Autodesk Fusion 360 part; units mm, degrees
note: some values were not read from the file. Set by a fixed rule: which face or edge a step refers to.
(part 3 of 3)
sketch "Skizze19" plane through (0, 0, 10) normal (0, 0, -1) x (1, 0, 0)
  circle A0 centre (420.5074, 124.379) radius 12
  circle A1 centre (87.5074, 162.379) radius 12
  circle A2 centre (120.8074, 162.379) radius 12
  circle A3 centre (154.1074, 162.379) radius 12
  circle A4 centre (187.4074, 162.379) radius 12
  circle A5 centre (220.7074, 162.379) radius 12
  circle A6 centre (254.0074, 162.379) radius 12
  circle A7 centre (287.3074, 162.379) radius 12
  circle A8 centre (320.6074, 162.379) radius 12
  circle A9 centre (353.9074, 162.379) radius 12
  circle A10 centre (387.2074, 162.379) radius 12
  circle A11 centre (420.5074, 162.379) radius 12
  line L0 (376.8151, 194.379) -> (364.2997, 194.379)
  arc A12 (343.5151, 194.379) -> (364.2997, 194.379) centre (353.9074, 200.379) ccw
  line L1 (343.5151, 194.379) -> (330.9997, 194.379)
  arc A13 (310.2151, 194.379) -> (330.9997, 194.379) centre (320.6074, 200.379) ccw
  line L2 (310.2151, 194.379) -> (297.6997, 194.379)
  arc A14 (276.9151, 194.379) -> (297.6997, 194.379) centre (287.3074, 200.379) ccw
  line L3 (276.9151, 194.379) -> (264.3997, 194.379)
  arc A15 (243.6151, 194.379) -> (264.3997, 194.379) centre (254.0074, 200.379) ccw
  line L4 (243.6151, 194.379) -> (231.0997, 194.379)
  arc A16 (210.3151, 194.379) -> (231.0997, 194.379) centre (220.7074, 200.379) ccw
  line L5 (210.3151, 194.379) -> (197.7997, 194.379)
  arc A17 (177.0151, 194.379) -> (197.7997, 194.379) centre (187.4074, 200.379) ccw
  line L6 (177.0151, 194.379) -> (164.4997, 194.379)
  arc A18 (143.7151, 194.379) -> (164.4997, 194.379) centre (154.1074, 200.379) ccw
  line L7 (143.7151, 194.379) -> (131.1997, 194.379)
  arc A19 (110.4151, 194.379) -> (131.1997, 194.379) centre (120.8074, 200.379) ccw
  line L8 (110.4151, 194.379) -> (97.8997, 194.379)
  arc A20 (77.1151, 194.379) -> (97.8997, 194.379) centre (87.5074, 200.379) ccw
  line L9 (77.1151, 194.379) -> (60.1074, 194.379)
  line L10 (60.1074, 194.379) -> (60.1074, 64.779)
  line L11 (60.1074, 64.779) -> (447.9074, 64.779)
  line L12 (447.9074, 64.779) -> (447.9074, 194.379)
  line L13 (447.9074, 194.379) -> (430.8997, 194.379)
  arc A21 (410.1151, 194.379) -> (430.8997, 194.379) centre (420.5074, 200.379) ccw
  line L14 (410.1151, 194.379) -> (397.5997, 194.379)
  arc A22 (376.8151, 194.379) -> (397.5997, 194.379) centre (387.2074, 200.379) ccw
  circle A23 centre (87.5074, 86.379) radius 12
  circle A24 centre (120.8074, 86.379) radius 12
  circle A25 centre (154.1074, 86.379) radius 12
  circle A26 centre (187.4074, 86.379) radius 12
  circle A27 centre (220.7074, 86.379) radius 12
  circle A28 centre (254.0074, 86.379) radius 12
  circle A29 centre (287.3074, 86.379) radius 12
  circle A30 centre (320.6074, 86.379) radius 12
  circle A31 centre (353.9074, 86.379) radius 12
  circle A32 centre (387.2074, 86.379) radius 12
  circle A33 centre (420.5074, 86.379) radius 12
  circle A34 centre (87.5074, 124.379) radius 12
  circle A35 centre (120.8074, 124.379) radius 12
  circle A36 centre (154.1074, 124.379) radius 12
  circle A37 centre (187.4074, 124.379) radius 12
  circle A38 centre (220.7074, 124.379) radius 12
  circle A39 centre (254.0074, 124.379) radius 12
  circle A40 centre (287.3074, 124.379) radius 12
  circle A41 centre (320.6074, 124.379) radius 12
  circle A42 centre (353.9074, 124.379) radius 12
  circle A43 centre (387.2074, 124.379) radius 12
  line L15 (60.1074, 168.379) -> (447.9074, 168.379)
  line L16 (447.9074, 168.379) -> (447.9074, 156.379)
  line L17 (447.9074, 156.379) -> (60.1074, 156.379)
  line L18 (60.1074, 156.379) -> (60.1074, 168.379)
  dimension "d256" = 6
  dimension "d257" = 6
  constraint horizontal L15
  constraint vertical L16
  constraint horizontal L17
  constraint vertical L18
  constraint collinear L10 L18
  constraint collinear L12 L16
  measures "d256" distance of A1.centre L15
  measures "d257" distance of A1.centre L17
extrude "Extrusion22" cut sketch "Skizze19" against normal blind 1 contours A1 A2 L15 L17 | A1 L10 L15 L17 L18 | A2 A3 L15 L17 | A3 A4 L15 L17 | A11 L12 L15 L16 L17 | A4 A5 L15 L17 | A10 A11 L15 L17 | A5 A6 L15 L17 | A9 A10 L15 L17 | A6 A7 L15 L17 | A8 A9 L15 L17 | A7 A8 L15 L17
sketch "Skizze20" plane through (0, 0, 10) normal (0, 0, -1) x (1, 0, 0)
  circle A0 centre (387.2074, 124.379) radius 12
  circle A1 centre (353.9074, 124.379) radius 12
  circle A2 centre (320.6074, 124.379) radius 12
  circle A3 centre (287.3074, 124.379) radius 12
  circle A4 centre (254.0074, 124.379) radius 12
  circle A5 centre (220.7074, 124.379) radius 12
  circle A6 centre (187.4074, 124.379) radius 12
  circle A7 centre (154.1074, 124.379) radius 12
  circle A8 centre (120.8074, 124.379) radius 12
  circle A9 centre (87.5074, 124.379) radius 12
  circle A10 centre (420.5074, 86.379) radius 12
  circle A11 centre (387.2074, 86.379) radius 12
  circle A12 centre (353.9074, 86.379) radius 12
  circle A13 centre (320.6074, 86.379) radius 12
  circle A14 centre (287.3074, 86.379) radius 12
  circle A15 centre (254.0074, 86.379) radius 12
  circle A16 centre (220.7074, 86.379) radius 12
  circle A17 centre (187.4074, 86.379) radius 12
  circle A18 centre (154.1074, 86.379) radius 12
  circle A19 centre (120.8074, 86.379) radius 12
  circle A20 centre (87.5074, 86.379) radius 12
  line L0 (376.8151, 156.379) -> (364.2997, 156.379)
  arc A21 (343.5151, 156.379) -> (364.2997, 156.379) centre (353.9074, 162.379) ccw
  line L1 (343.5151, 156.379) -> (330.9997, 156.379)
  arc A22 (310.2151, 156.379) -> (330.9997, 156.379) centre (320.6074, 162.379) ccw
  line L2 (310.2151, 156.379) -> (297.6997, 156.379)
  arc A23 (276.9151, 156.379) -> (297.6997, 156.379) centre (287.3074, 162.379) ccw
  line L3 (276.9151, 156.379) -> (264.3997, 156.379)
  arc A24 (243.6151, 156.379) -> (264.3997, 156.379) centre (254.0074, 162.379) ccw
  line L4 (243.6151, 156.379) -> (231.0997, 156.379)
  arc A25 (210.3151, 156.379) -> (231.0997, 156.379) centre (220.7074, 162.379) ccw
  line L5 (210.3151, 156.379) -> (197.7997, 156.379)
  arc A26 (177.0151, 156.379) -> (197.7997, 156.379) centre (187.4074, 162.379) ccw
  line L6 (177.0151, 156.379) -> (164.4997, 156.379)
  arc A27 (143.7151, 156.379) -> (164.4997, 156.379) centre (154.1074, 162.379) ccw
  line L7 (143.7151, 156.379) -> (131.1997, 156.379)
  arc A28 (110.4151, 156.379) -> (131.1997, 156.379) centre (120.8074, 162.379) ccw
  line L8 (110.4151, 156.379) -> (97.8997, 156.379)
  arc A29 (77.1151, 156.379) -> (97.8997, 156.379) centre (87.5074, 162.379) ccw
  line L9 (77.1151, 156.379) -> (60.1074, 156.379)
  line L10 (60.1074, 156.379) -> (60.1074, 64.779)
  line L11 (60.1074, 64.779) -> (447.9074, 64.779)
  line L12 (447.9074, 64.779) -> (447.9074, 156.379)
  line L13 (447.9074, 156.379) -> (430.8997, 156.379)
  arc A30 (410.1151, 156.379) -> (430.8997, 156.379) centre (420.5074, 162.379) ccw
  line L14 (410.1151, 156.379) -> (397.5997, 156.379)
  arc A31 (376.8151, 156.379) -> (397.5997, 156.379) centre (387.2074, 162.379) ccw
  circle A32 centre (420.5074, 124.379) radius 12
  line L15 (60.1074, 130.379) -> (447.9074, 130.379)
  line L16 (447.9074, 130.379) -> (447.9074, 118.379)
  line L17 (447.9074, 118.379) -> (60.1074, 118.379)
  line L18 (60.1074, 118.379) -> (60.1074, 130.379)
  dimension "d260" = 6
  dimension "d261" = 6
  constraint horizontal L15
  constraint vertical L16
  constraint horizontal L17
  constraint vertical L18
  constraint collinear L10 L18
  constraint collinear L12 L16
  measures "d260" distance of A9.centre L15
  measures "d261" distance of A9.centre L17
extrude "Extrusion23" cut sketch "Skizze20" against normal blind 1 contours A0 A32 L15 L17 | A0 A1 L15 L17 | L12 A32 L15 L16 L17 | A1 A2 L15 L17 | A2 A3 L15 L17 | A9 L10 L15 L17 L18 | A3 A4 L15 L17 | A8 A9 L15 L17 | A4 A5 L15 L17 | A7 A8 L15 L17 | A5 A6 L15 L17 | A6 A7 L15 L17
sketch "Skizze21" plane through (0, 0, 10) normal (0, 0, -1) x (1, 0, 0)
  circle A0 centre (87.5074, 86.379) radius 12
  circle A1 centre (120.8074, 86.379) radius 12
  circle A2 centre (154.1074, 86.379) radius 12
  circle A3 centre (187.4074, 86.379) radius 12
  circle A4 centre (220.7074, 86.379) radius 12
  circle A5 centre (254.0074, 86.379) radius 12
  circle A6 centre (287.3074, 86.379) radius 12
  circle A7 centre (320.6074, 86.379) radius 12
  circle A8 centre (353.9074, 86.379) radius 12
  circle A9 centre (387.2074, 86.379) radius 12
  circle A10 centre (420.5074, 86.379) radius 12
  line L0 (376.8151, 118.379) -> (364.2997, 118.379)
  arc A11 (343.5151, 118.379) -> (364.2997, 118.379) centre (353.9074, 124.379) ccw
  line L1 (343.5151, 118.379) -> (330.9997, 118.379)
  arc A12 (310.2151, 118.379) -> (330.9997, 118.379) centre (320.6074, 124.379) ccw
  line L2 (310.2151, 118.379) -> (297.6997, 118.379)
  arc A13 (276.9151, 118.379) -> (297.6997, 118.379) centre (287.3074, 124.379) ccw
  line L3 (276.9151, 118.379) -> (264.3997, 118.379)
  arc A14 (243.6151, 118.379) -> (264.3997, 118.379) centre (254.0074, 124.379) ccw
  line L4 (243.6151, 118.379) -> (231.0997, 118.379)
  arc A15 (210.3151, 118.379) -> (231.0997, 118.379) centre (220.7074, 124.379) ccw
  line L5 (210.3151, 118.379) -> (197.7997, 118.379)
  arc A16 (177.0151, 118.379) -> (197.7997, 118.379) centre (187.4074, 124.379) ccw
  line L6 (177.0151, 118.379) -> (164.4997, 118.379)
  arc A17 (143.7151, 118.379) -> (164.4997, 118.379) centre (154.1074, 124.379) ccw
  line L7 (143.7151, 118.379) -> (131.1997, 118.379)
  arc A18 (110.4151, 118.379) -> (131.1997, 118.379) centre (120.8074, 124.379) ccw
  line L8 (110.4151, 118.379) -> (97.8997, 118.379)
  arc A19 (77.1151, 118.379) -> (97.8997, 118.379) centre (87.5074, 124.379) ccw
  line L9 (77.1151, 118.379) -> (60.1074, 118.379)
  line L10 (60.1074, 118.379) -> (60.1074, 64.779)
  line L11 (60.1074, 64.779) -> (447.9074, 64.779)
  line L12 (447.9074, 64.779) -> (447.9074, 118.379)
  line L13 (447.9074, 118.379) -> (430.8997, 118.379)
  arc A20 (410.1151, 118.379) -> (430.8997, 118.379) centre (420.5074, 124.379) ccw
  line L14 (410.1151, 118.379) -> (397.5997, 118.379)
  arc A21 (376.8151, 118.379) -> (397.5997, 118.379) centre (387.2074, 124.379) ccw
  line L15 (60.1074, 92.379) -> (447.9074, 92.379)
  line L16 (447.9074, 92.379) -> (447.9074, 80.379)
  line L17 (447.9074, 80.379) -> (60.1074, 80.379)
  line L18 (60.1074, 80.379) -> (60.1074, 92.379)
  dimension "d264" = 6
  dimension "d265" = 6
  constraint horizontal L15
  constraint vertical L16
  constraint horizontal L17
  constraint vertical L18
  constraint collinear L10 L18
  constraint collinear L12 L16
  measures "d264" distance of A0.centre L15
  measures "d265" distance of A0.centre L17
extrude "Extrusion24" cut sketch "Skizze21" against normal blind 1 contours A0 A1 L15 L17 | A0 L10 L15 L17 L18 | A1 A2 L15 L17 | A2 A3 L15 L17 | A10 L12 L15 L16 L17 | A3 A4 L15 L17 | A9 A10 L15 L17 | A4 A5 L15 L17 | A8 A9 L15 L17 | A5 A6 L15 L17 | A7 A8 L15 L17 | A6 A7 L15 L17
sketch "Skizze22" plane through (0, 0, 30) normal (0, 0, 1) x (-1, 0, 0)
  circle A0 centre (-120.8074, 276.379) radius 12
  circle A1 centre (-87.5074, 276.379) radius 12
  circle A2 centre (-420.5074, 238.379) radius 12
  circle A3 centre (-387.2074, 238.379) radius 12
  circle A4 centre (-87.5074, 86.379) radius 12
  circle A5 centre (-28.1074, 23.779) radius 10.8095
  circle A6 centre (-479.9074, 23.779) radius 12
  circle A7 centre (-120.8074, 86.379) radius 12
  circle A8 centre (-154.1074, 86.379) radius 12
  circle A9 centre (-187.4074, 86.379) radius 12
  circle A10 centre (-220.7074, 86.379) radius 12
  circle A11 centre (-254.0074, 86.379) radius 12
  circle A12 centre (-287.3074, 86.379) radius 12
  circle A13 centre (-320.6074, 86.379) radius 12
  circle A14 centre (-353.9074, 86.379) radius 12
  circle A15 centre (-387.2074, 86.379) radius 12
  circle A16 centre (-120.8074, 124.379) radius 12
  circle A17 centre (-220.7074, 124.379) radius 12
  circle A18 centre (-320.6074, 124.379) radius 12
  circle A19 centre (-353.9074, 124.379) radius 12
  circle A20 centre (-254.0074, 124.379) radius 12
  circle A21 centre (-154.1074, 124.379) radius 12
  circle A22 centre (-420.5074, 86.379) radius 12
  circle A23 centre (-87.5074, 124.379) radius 12
  circle A24 centre (-187.4074, 124.379) radius 12
  circle A25 centre (-287.3074, 124.379) radius 12
  circle A26 centre (-387.2074, 124.379) radius 12
  circle A27 centre (-387.2074, 276.379) radius 12
  circle A28 centre (-87.5074, 314.379) radius 12
  circle A29 centre (-320.6074, 314.379) radius 12
  circle A30 centre (-120.8074, 314.379) radius 12
  circle A31 centre (-187.4074, 276.379) radius 12
  circle A32 centre (-353.9074, 276.379) radius 12
  circle A33 centre (-287.3074, 314.379) radius 12
  circle A34 centre (-154.1074, 314.379) radius 12
  circle A35 centre (-220.7074, 276.379) radius 12
  circle A36 centre (-320.6074, 276.379) radius 12
  circle A37 centre (-254.0074, 314.379) radius 12
  circle A38 centre (-187.4074, 314.379) radius 12
  circle A39 centre (-254.0074, 276.379) radius 12
  circle A40 centre (-120.8074, 352.379) radius 12
  circle A41 centre (-187.4074, 238.379) radius 12
  circle A42 centre (-387.2074, 200.379) radius 12
  circle A43 centre (-220.7074, 200.379) radius 12
  circle A44 centre (-420.5074, 162.379) radius 12
  circle A45 centre (-254.0074, 162.379) radius 12
  circle A46 centre (-87.5074, 162.379) radius 12
  circle A47 centre (-420.5074, 352.379) radius 12
  circle A48 centre (-220.7074, 390.379) radius 12
  circle A49 centre (-187.4074, 390.379) radius 12
  circle A50 centre (-387.2074, 352.379) radius 12
  circle A51 centre (-120.8074, 162.379) radius 12
  circle A52 centre (-287.3074, 162.379) radius 12
  circle A53 centre (-87.5074, 200.379) radius 12
  circle A54 centre (-254.0074, 200.379) radius 12
  circle A55 centre (-420.5074, 200.379) radius 12
  circle A56 centre (-220.7074, 238.379) radius 12
  circle A57 centre (-254.0074, 238.379) radius 12
  circle A58 centre (-287.3074, 238.379) radius 12
  circle A59 centre (-320.6074, 238.379) radius 12
  circle A60 centre (-353.9074, 238.379) radius 12
  circle A61 centre (-254.0074, 352.379) radius 12
  circle A62 centre (-87.5074, 352.379) radius 12
  circle A63 centre (-420.5074, 314.379) radius 12
  circle A64 centre (-220.7074, 314.379) radius 12
  circle A65 centre (-287.3074, 276.379) radius 12
  circle A66 centre (-220.7074, 352.379) radius 12
  circle A67 centre (-87.5074, 238.379) radius 12
  circle A68 centre (-287.3074, 200.379) radius 12
  circle A69 centre (-120.8074, 200.379) radius 12
  circle A70 centre (-320.6074, 162.379) radius 12
  circle A71 centre (-154.1074, 162.379) radius 12
  circle A72 centre (-353.9074, 352.379) radius 12
  circle A73 centre (-154.1074, 390.379) radius 12
  circle A74 centre (-320.6074, 390.379) radius 12
  circle A75 centre (-353.9074, 390.379) radius 12
  circle A76 centre (-387.2074, 390.379) radius 12
  circle A77 centre (-420.5074, 390.379) radius 12
  circle A78 centre (-87.5074, 428.379) radius 12
  circle A79 centre (-120.8074, 428.379) radius 12
  circle A80 centre (-154.1074, 428.379) radius 12
  circle A81 centre (-187.4074, 428.379) radius 12
  circle A82 centre (-220.7074, 428.379) radius 12
  circle A83 centre (-254.0074, 428.379) radius 12
  circle A84 centre (-287.3074, 428.379) radius 12
  circle A85 centre (-320.6074, 428.379) radius 12
  circle A86 centre (-353.9074, 428.379) radius 12
  circle A87 centre (-387.2074, 428.379) radius 12
  circle A88 centre (-420.5074, 428.379) radius 12
  circle A89 centre (-28.1074, 490.979) radius 12
  circle A90 centre (-287.3074, 390.379) radius 12
  circle A91 centre (-120.8074, 390.379) radius 12
  circle A92 centre (-320.6074, 352.379) radius 12
  circle A93 centre (-187.4074, 162.379) radius 12
  circle A94 centre (-353.9074, 162.379) radius 12
  circle A95 centre (-154.1074, 200.379) radius 12
  circle A96 centre (-320.6074, 200.379) radius 12
  circle A97 centre (-120.8074, 238.379) radius 12
  circle A98 centre (-187.4074, 352.379) radius 12
  circle A99 centre (-154.1074, 352.379) radius 12
  circle A100 centre (-387.2074, 314.379) radius 12
  circle A101 centre (-154.1074, 238.379) radius 12
  circle A102 centre (-353.9074, 200.379) radius 12
  circle A103 centre (-187.4074, 200.379) radius 12
  circle A104 centre (-387.2074, 162.379) radius 12
  circle A105 centre (-420.5074, 276.379) radius 12
  circle A106 centre (-154.1074, 276.379) radius 12
  circle A107 centre (-220.7074, 162.379) radius 12
  circle A108 centre (-353.9074, 314.379) radius 12
  circle A109 centre (-420.5074, 124.379) radius 12
  circle A110 centre (-87.5074, 390.379) radius 12
  circle A111 centre (-254.0074, 390.379) radius 12
  circle A112 centre (-479.9074, 490.979) radius 12
  circle A113 centre (-287.3074, 352.379) radius 12
  line L0 (-0.1074, -0.221) -> (-0.1074, 514.979)
  line L1 (-0.1074, 514.979) -> (-507.9074, 514.979)
  line L2 (-507.9074, 514.979) -> (-507.9074, -0.221)
  line L3 (-507.9074, -0.221) -> (-0.1074, -0.221)
  circle A114 centre (-50.1074, 49.779) radius 7.5
  dimension "d268" = 15
  dimension "d269" = 50
  dimension "d270" = 50
  measures "d268" diameter of A114
  measures "d269" distance of L0 A114.centre
  measures "d270" distance of L3 A114.centre
extrude "Extrusion25" cut sketch "Skizze22" against normal blind 4 contours A114
sketch "Skizze23" plane through (0, 0, 30) normal (0, 0, 1) x (-1, 0, 0)
  circle A0 centre (-50.1074, 49.779) radius 7.5
  circle A1 centre (-120.8074, 276.379) radius 12
  circle A2 centre (-87.5074, 276.379) radius 12
  circle A3 centre (-420.5074, 238.379) radius 12
  circle A4 centre (-387.2074, 238.379) radius 12
  circle A5 centre (-87.5074, 86.379) radius 12
  circle A6 centre (-28.1074, 23.779) radius 10.8095
  circle A7 centre (-479.9074, 23.779) radius 12
  circle A8 centre (-120.8074, 86.379) radius 12
  circle A9 centre (-154.1074, 86.379) radius 12
  circle A10 centre (-187.4074, 86.379) radius 12
  circle A11 centre (-220.7074, 86.379) radius 12
  circle A12 centre (-254.0074, 86.379) radius 12
  circle A13 centre (-287.3074, 86.379) radius 12
  circle A14 centre (-320.6074, 86.379) radius 12
  circle A15 centre (-353.9074, 86.379) radius 12
  circle A16 centre (-387.2074, 86.379) radius 12
  circle A17 centre (-120.8074, 124.379) radius 12
  circle A18 centre (-220.7074, 124.379) radius 12
  circle A19 centre (-320.6074, 124.379) radius 12
  circle A20 centre (-353.9074, 124.379) radius 12
  circle A21 centre (-254.0074, 124.379) radius 12
  circle A22 centre (-154.1074, 124.379) radius 12
  circle A23 centre (-420.5074, 86.379) radius 12
  circle A24 centre (-87.5074, 124.379) radius 12
  circle A25 centre (-187.4074, 124.379) radius 12
  circle A26 centre (-287.3074, 124.379) radius 12
  circle A27 centre (-387.2074, 124.379) radius 12
  circle A28 centre (-387.2074, 276.379) radius 12
  circle A29 centre (-87.5074, 314.379) radius 12
  circle A30 centre (-320.6074, 314.379) radius 12
  circle A31 centre (-120.8074, 314.379) radius 12
  circle A32 centre (-187.4074, 276.379) radius 12
  circle A33 centre (-353.9074, 276.379) radius 12
  circle A34 centre (-287.3074, 314.379) radius 12
  circle A35 centre (-154.1074, 314.379) radius 12
  circle A36 centre (-220.7074, 276.379) radius 12
  circle A37 centre (-320.6074, 276.379) radius 12
  circle A38 centre (-254.0074, 314.379) radius 12
  circle A39 centre (-187.4074, 314.379) radius 12
  circle A40 centre (-254.0074, 276.379) radius 12
  circle A41 centre (-120.8074, 352.379) radius 12
  circle A42 centre (-187.4074, 238.379) radius 12
  circle A43 centre (-387.2074, 200.379) radius 12
  circle A44 centre (-220.7074, 200.379) radius 12
  circle A45 centre (-420.5074, 162.379) radius 12
  circle A46 centre (-254.0074, 162.379) radius 12
  circle A47 centre (-87.5074, 162.379) radius 12
  circle A48 centre (-420.5074, 352.379) radius 12
  circle A49 centre (-220.7074, 390.379) radius 12
  circle A50 centre (-187.4074, 390.379) radius 12
  circle A51 centre (-387.2074, 352.379) radius 12
  circle A52 centre (-120.8074, 162.379) radius 12
  circle A53 centre (-287.3074, 162.379) radius 12
  circle A54 centre (-87.5074, 200.379) radius 12
  circle A55 centre (-254.0074, 200.379) radius 12
  circle A56 centre (-420.5074, 200.379) radius 12
  circle A57 centre (-220.7074, 238.379) radius 12
  circle A58 centre (-254.0074, 238.379) radius 12
  circle A59 centre (-287.3074, 238.379) radius 12
  circle A60 centre (-320.6074, 238.379) radius 12
  circle A61 centre (-353.9074, 238.379) radius 12
  circle A62 centre (-254.0074, 352.379) radius 12
  circle A63 centre (-87.5074, 352.379) radius 12
  circle A64 centre (-420.5074, 314.379) radius 12
  circle A65 centre (-220.7074, 314.379) radius 12
  circle A66 centre (-287.3074, 276.379) radius 12
  circle A67 centre (-220.7074, 352.379) radius 12
  circle A68 centre (-87.5074, 238.379) radius 12
  circle A69 centre (-287.3074, 200.379) radius 12
  circle A70 centre (-120.8074, 200.379) radius 12
  circle A71 centre (-320.6074, 162.379) radius 12
  circle A72 centre (-154.1074, 162.379) radius 12
  circle A73 centre (-353.9074, 352.379) radius 12
  circle A74 centre (-154.1074, 390.379) radius 12
  circle A75 centre (-320.6074, 390.379) radius 12
  circle A76 centre (-353.9074, 390.379) radius 12
  circle A77 centre (-387.2074, 390.379) radius 12
  circle A78 centre (-420.5074, 390.379) radius 12
  circle A79 centre (-87.5074, 428.379) radius 12
  circle A80 centre (-120.8074, 428.379) radius 12
  circle A81 centre (-154.1074, 428.379) radius 12
  circle A82 centre (-187.4074, 428.379) radius 12
  circle A83 centre (-220.7074, 428.379) radius 12
  circle A84 centre (-254.0074, 428.379) radius 12
  circle A85 centre (-287.3074, 428.379) radius 12
  circle A86 centre (-320.6074, 428.379) radius 12
  circle A87 centre (-353.9074, 428.379) radius 12
  circle A88 centre (-387.2074, 428.379) radius 12
  circle A89 centre (-420.5074, 428.379) radius 12
  circle A90 centre (-28.1074, 490.979) radius 12
  circle A91 centre (-287.3074, 390.379) radius 12
  circle A92 centre (-120.8074, 390.379) radius 12
  circle A93 centre (-320.6074, 352.379) radius 12
  circle A94 centre (-187.4074, 162.379) radius 12
  circle A95 centre (-353.9074, 162.379) radius 12
  circle A96 centre (-154.1074, 200.379) radius 12
  circle A97 centre (-320.6074, 200.379) radius 12
  circle A98 centre (-120.8074, 238.379) radius 12
  circle A99 centre (-187.4074, 352.379) radius 12
  circle A100 centre (-154.1074, 352.379) radius 12
  circle A101 centre (-387.2074, 314.379) radius 12
  circle A102 centre (-154.1074, 238.379) radius 12
  circle A103 centre (-353.9074, 200.379) radius 12
  circle A104 centre (-187.4074, 200.379) radius 12
  circle A105 centre (-387.2074, 162.379) radius 12
  circle A106 centre (-420.5074, 276.379) radius 12
  circle A107 centre (-154.1074, 276.379) radius 12
  circle A108 centre (-220.7074, 162.379) radius 12
  circle A109 centre (-353.9074, 314.379) radius 12
  circle A110 centre (-420.5074, 124.379) radius 12
  circle A111 centre (-87.5074, 390.379) radius 12
  circle A112 centre (-254.0074, 390.379) radius 12
  circle A113 centre (-479.9074, 490.979) radius 12
  circle A114 centre (-287.3074, 352.379) radius 12
  line L0 (-0.1074, -0.221) -> (-0.1074, 514.979)
  line L1 (-0.1074, 514.979) -> (-507.9074, 514.979)
  line L2 (-507.9074, 514.979) -> (-507.9074, -0.221)
  line L3 (-507.9074, -0.221) -> (-0.1074, -0.221)
  circle A115 centre (-457.9074, 49.779) radius 7.5
  dimension "d273" = 15
  dimension "d274" = 50
  dimension "d275" = 50
  measures "d273" diameter of A115
  measures "d274" distance of L3 A115.centre
  measures "d275" distance of L2 A115.centre
extrude "Extrusion26" cut sketch "Skizze23" against normal blind 4 contours A115
sketch "Skizze24" plane through (0, 0, 30) normal (0, 0, 1) x (-1, 0, 0)
  circle A0 centre (-457.9074, 49.779) radius 7.5
  circle A1 centre (-50.1074, 49.779) radius 7.5
  circle A2 centre (-120.8074, 276.379) radius 12
  circle A3 centre (-87.5074, 276.379) radius 12
  circle A4 centre (-420.5074, 238.379) radius 12
  circle A5 centre (-387.2074, 238.379) radius 12
  circle A6 centre (-87.5074, 86.379) radius 12
  circle A7 centre (-28.1074, 23.779) radius 10.8095
  circle A8 centre (-479.9074, 23.779) radius 12
  circle A9 centre (-120.8074, 86.379) radius 12
  circle A10 centre (-154.1074, 86.379) radius 12
  circle A11 centre (-187.4074, 86.379) radius 12
  circle A12 centre (-220.7074, 86.379) radius 12
  circle A13 centre (-254.0074, 86.379) radius 12
  circle A14 centre (-287.3074, 86.379) radius 12
  circle A15 centre (-320.6074, 86.379) radius 12
  circle A16 centre (-353.9074, 86.379) radius 12
  circle A17 centre (-387.2074, 86.379) radius 12
  circle A18 centre (-120.8074, 124.379) radius 12
  circle A19 centre (-220.7074, 124.379) radius 12
  circle A20 centre (-320.6074, 124.379) radius 12
  circle A21 centre (-353.9074, 124.379) radius 12
  circle A22 centre (-254.0074, 124.379) radius 12
  circle A23 centre (-154.1074, 124.379) radius 12
  circle A24 centre (-420.5074, 86.379) radius 12
  circle A25 centre (-87.5074, 124.379) radius 12
  circle A26 centre (-187.4074, 124.379) radius 12
  circle A27 centre (-287.3074, 124.379) radius 12
  circle A28 centre (-387.2074, 124.379) radius 12
  circle A29 centre (-387.2074, 276.379) radius 12
  circle A30 centre (-87.5074, 314.379) radius 12
  circle A31 centre (-320.6074, 314.379) radius 12
  circle A32 centre (-120.8074, 314.379) radius 12
  circle A33 centre (-187.4074, 276.379) radius 12
  circle A34 centre (-353.9074, 276.379) radius 12
  circle A35 centre (-287.3074, 314.379) radius 12
  circle A36 centre (-154.1074, 314.379) radius 12
  circle A37 centre (-220.7074, 276.379) radius 12
  circle A38 centre (-320.6074, 276.379) radius 12
  circle A39 centre (-254.0074, 314.379) radius 12
  circle A40 centre (-187.4074, 314.379) radius 12
  circle A41 centre (-254.0074, 276.379) radius 12
  circle A42 centre (-120.8074, 352.379) radius 12
  circle A43 centre (-187.4074, 238.379) radius 12
  circle A44 centre (-387.2074, 200.379) radius 12
  circle A45 centre (-220.7074, 200.379) radius 12
  circle A46 centre (-420.5074, 162.379) radius 12
  circle A47 centre (-254.0074, 162.379) radius 12
  circle A48 centre (-87.5074, 162.379) radius 12
  circle A49 centre (-420.5074, 352.379) radius 12
  circle A50 centre (-220.7074, 390.379) radius 12
  circle A51 centre (-187.4074, 390.379) radius 12
  circle A52 centre (-387.2074, 352.379) radius 12
  circle A53 centre (-120.8074, 162.379) radius 12
  circle A54 centre (-287.3074, 162.379) radius 12
  circle A55 centre (-87.5074, 200.379) radius 12
  circle A56 centre (-254.0074, 200.379) radius 12
  circle A57 centre (-420.5074, 200.379) radius 12
  circle A58 centre (-220.7074, 238.379) radius 12
  circle A59 centre (-254.0074, 238.379) radius 12
  circle A60 centre (-287.3074, 238.379) radius 12
  circle A61 centre (-320.6074, 238.379) radius 12
  circle A62 centre (-353.9074, 238.379) radius 12
  circle A63 centre (-254.0074, 352.379) radius 12
  circle A64 centre (-87.5074, 352.379) radius 12
  circle A65 centre (-420.5074, 314.379) radius 12
  circle A66 centre (-220.7074, 314.379) radius 12
  circle A67 centre (-287.3074, 276.379) radius 12
  circle A68 centre (-220.7074, 352.379) radius 12
  circle A69 centre (-87.5074, 238.379) radius 12
  circle A70 centre (-287.3074, 200.379) radius 12
  circle A71 centre (-120.8074, 200.379) radius 12
  circle A72 centre (-320.6074, 162.379) radius 12
  circle A73 centre (-154.1074, 162.379) radius 12
  circle A74 centre (-353.9074, 352.379) radius 12
  circle A75 centre (-154.1074, 390.379) radius 12
  circle A76 centre (-320.6074, 390.379) radius 12
  circle A77 centre (-353.9074, 390.379) radius 12
  circle A78 centre (-387.2074, 390.379) radius 12
  circle A79 centre (-420.5074, 390.379) radius 12
  circle A80 centre (-87.5074, 428.379) radius 12
  circle A81 centre (-120.8074, 428.379) radius 12
  circle A82 centre (-154.1074, 428.379) radius 12
  circle A83 centre (-187.4074, 428.379) radius 12
  circle A84 centre (-220.7074, 428.379) radius 12
  circle A85 centre (-254.0074, 428.379) radius 12
  circle A86 centre (-287.3074, 428.379) radius 12
  circle A87 centre (-320.6074, 428.379) radius 12
  circle A88 centre (-353.9074, 428.379) radius 12
  circle A89 centre (-387.2074, 428.379) radius 12
  circle A90 centre (-420.5074, 428.379) radius 12
  circle A91 centre (-28.1074, 490.979) radius 12
  circle A92 centre (-287.3074, 390.379) radius 12
  circle A93 centre (-120.8074, 390.379) radius 12
  circle A94 centre (-320.6074, 352.379) radius 12
  circle A95 centre (-187.4074, 162.379) radius 12
  circle A96 centre (-353.9074, 162.379) radius 12
  circle A97 centre (-154.1074, 200.379) radius 12
  circle A98 centre (-320.6074, 200.379) radius 12
  circle A99 centre (-120.8074, 238.379) radius 12
  circle A100 centre (-187.4074, 352.379) radius 12
  circle A101 centre (-154.1074, 352.379) radius 12
  circle A102 centre (-387.2074, 314.379) radius 12
  circle A103 centre (-154.1074, 238.379) radius 12
  circle A104 centre (-353.9074, 200.379) radius 12
  circle A105 centre (-187.4074, 200.379) radius 12
  circle A106 centre (-387.2074, 162.379) radius 12
  circle A107 centre (-420.5074, 276.379) radius 12
  circle A108 centre (-154.1074, 276.379) radius 12
  circle A109 centre (-220.7074, 162.379) radius 12
  circle A110 centre (-353.9074, 314.379) radius 12
  circle A111 centre (-420.5074, 124.379) radius 12
  circle A112 centre (-87.5074, 390.379) radius 12
  circle A113 centre (-254.0074, 390.379) radius 12
  circle A114 centre (-479.9074, 490.979) radius 12
  circle A115 centre (-287.3074, 352.379) radius 12
  line L0 (-0.1074, -0.221) -> (-0.1074, 514.979)
  line L1 (-0.1074, 514.979) -> (-507.9074, 514.979)
  line L2 (-507.9074, 514.979) -> (-507.9074, -0.221)
  line L3 (-507.9074, -0.221) -> (-0.1074, -0.221)
  circle A116 centre (-457.9074, 464.979) radius 7.5
  dimension "d278" = 15
  dimension "d279" = 50
  dimension "d280" = 50
  measures "d278" diameter of A116
  measures "d279" distance of L2 A116.centre
  measures "d280" distance of L1 A116.centre
extrude "Extrusion27" cut sketch "Skizze24" against normal blind 4 contours A116
sketch "Skizze25" plane through (0, 0, 30) normal (0, 0, 1) x (-1, 0, 0)
  circle A0 centre (-457.9074, 464.979) radius 7.5
  circle A1 centre (-457.9074, 49.779) radius 7.5
  circle A2 centre (-50.1074, 49.779) radius 7.5
  circle A3 centre (-120.8074, 276.379) radius 12
  circle A4 centre (-87.5074, 276.379) radius 12
  circle A5 centre (-420.5074, 238.379) radius 12
  circle A6 centre (-387.2074, 238.379) radius 12
  circle A7 centre (-87.5074, 86.379) radius 12
  circle A8 centre (-28.1074, 23.779) radius 10.8095
  circle A9 centre (-479.9074, 23.779) radius 12
  circle A10 centre (-120.8074, 86.379) radius 12
  circle A11 centre (-154.1074, 86.379) radius 12
  circle A12 centre (-187.4074, 86.379) radius 12
  circle A13 centre (-220.7074, 86.379) radius 12
  circle A14 centre (-254.0074, 86.379) radius 12
  circle A15 centre (-287.3074, 86.379) radius 12
  circle A16 centre (-320.6074, 86.379) radius 12
  circle A17 centre (-353.9074, 86.379) radius 12
  circle A18 centre (-387.2074, 86.379) radius 12
  circle A19 centre (-120.8074, 124.379) radius 12
  circle A20 centre (-220.7074, 124.379) radius 12
  circle A21 centre (-320.6074, 124.379) radius 12
  circle A22 centre (-353.9074, 124.379) radius 12
  circle A23 centre (-254.0074, 124.379) radius 12
  circle A24 centre (-154.1074, 124.379) radius 12
  circle A25 centre (-420.5074, 86.379) radius 12
  circle A26 centre (-87.5074, 124.379) radius 12
  circle A27 centre (-187.4074, 124.379) radius 12
  circle A28 centre (-287.3074, 124.379) radius 12
  circle A29 centre (-387.2074, 124.379) radius 12
  circle A30 centre (-387.2074, 276.379) radius 12
  circle A31 centre (-87.5074, 314.379) radius 12
  circle A32 centre (-320.6074, 314.379) radius 12
  circle A33 centre (-120.8074, 314.379) radius 12
  circle A34 centre (-187.4074, 276.379) radius 12
  circle A35 centre (-353.9074, 276.379) radius 12
  circle A36 centre (-287.3074, 314.379) radius 12
  circle A37 centre (-154.1074, 314.379) radius 12
  circle A38 centre (-220.7074, 276.379) radius 12
  circle A39 centre (-320.6074, 276.379) radius 12
  circle A40 centre (-254.0074, 314.379) radius 12
  circle A41 centre (-187.4074, 314.379) radius 12
  circle A42 centre (-254.0074, 276.379) radius 12
  circle A43 centre (-120.8074, 352.379) radius 12
  circle A44 centre (-187.4074, 238.379) radius 12
  circle A45 centre (-387.2074, 200.379) radius 12
  circle A46 centre (-220.7074, 200.379) radius 12
  circle A47 centre (-420.5074, 162.379) radius 12
  circle A48 centre (-254.0074, 162.379) radius 12
  circle A49 centre (-87.5074, 162.379) radius 12
  circle A50 centre (-420.5074, 352.379) radius 12
  circle A51 centre (-220.7074, 390.379) radius 12
  circle A52 centre (-187.4074, 390.379) radius 12
  circle A53 centre (-387.2074, 352.379) radius 12
  circle A54 centre (-120.8074, 162.379) radius 12
  circle A55 centre (-287.3074, 162.379) radius 12
  circle A56 centre (-87.5074, 200.379) radius 12
  circle A57 centre (-254.0074, 200.379) radius 12
  circle A58 centre (-420.5074, 200.379) radius 12
  circle A59 centre (-220.7074, 238.379) radius 12
  circle A60 centre (-254.0074, 238.379) radius 12
  circle A61 centre (-287.3074, 238.379) radius 12
  circle A62 centre (-320.6074, 238.379) radius 12
  circle A63 centre (-353.9074, 238.379) radius 12
  circle A64 centre (-254.0074, 352.379) radius 12
  circle A65 centre (-87.5074, 352.379) radius 12
  circle A66 centre (-420.5074, 314.379) radius 12
  circle A67 centre (-220.7074, 314.379) radius 12
  circle A68 centre (-287.3074, 276.379) radius 12
  circle A69 centre (-220.7074, 352.379) radius 12
  circle A70 centre (-87.5074, 238.379) radius 12
  circle A71 centre (-287.3074, 200.379) radius 12
  circle A72 centre (-120.8074, 200.379) radius 12
  circle A73 centre (-320.6074, 162.379) radius 12
  circle A74 centre (-154.1074, 162.379) radius 12
  circle A75 centre (-353.9074, 352.379) radius 12
  circle A76 centre (-154.1074, 390.379) radius 12
  circle A77 centre (-320.6074, 390.379) radius 12
  circle A78 centre (-353.9074, 390.379) radius 12
  circle A79 centre (-387.2074, 390.379) radius 12
  circle A80 centre (-420.5074, 390.379) radius 12
  circle A81 centre (-87.5074, 428.379) radius 12
  circle A82 centre (-120.8074, 428.379) radius 12
  circle A83 centre (-154.1074, 428.379) radius 12
  circle A84 centre (-187.4074, 428.379) radius 12
  circle A85 centre (-220.7074, 428.379) radius 12
  circle A86 centre (-254.0074, 428.379) radius 12
  circle A87 centre (-287.3074, 428.379) radius 12
  circle A88 centre (-320.6074, 428.379) radius 12
  circle A89 centre (-353.9074, 428.379) radius 12
  circle A90 centre (-387.2074, 428.379) radius 12
  circle A91 centre (-420.5074, 428.379) radius 12
  circle A92 centre (-28.1074, 490.979) radius 12
  circle A93 centre (-287.3074, 390.379) radius 12
  circle A94 centre (-120.8074, 390.379) radius 12
  circle A95 centre (-320.6074, 352.379) radius 12
  circle A96 centre (-187.4074, 162.379) radius 12
  circle A97 centre (-353.9074, 162.379) radius 12
  circle A98 centre (-154.1074, 200.379) radius 12
  circle A99 centre (-320.6074, 200.379) radius 12
  circle A100 centre (-120.8074, 238.379) radius 12
  circle A101 centre (-187.4074, 352.379) radius 12
  circle A102 centre (-154.1074, 352.379) radius 12
  circle A103 centre (-387.2074, 314.379) radius 12
  circle A104 centre (-154.1074, 238.379) radius 12
  circle A105 centre (-353.9074, 200.379) radius 12
  circle A106 centre (-187.4074, 200.379) radius 12
  circle A107 centre (-387.2074, 162.379) radius 12
  circle A108 centre (-420.5074, 276.379) radius 12
  circle A109 centre (-154.1074, 276.379) radius 12
  circle A110 centre (-220.7074, 162.379) radius 12
  circle A111 centre (-353.9074, 314.379) radius 12
  circle A112 centre (-420.5074, 124.379) radius 12
  circle A113 centre (-87.5074, 390.379) radius 12
  circle A114 centre (-254.0074, 390.379) radius 12
  circle A115 centre (-479.9074, 490.979) radius 12
  circle A116 centre (-287.3074, 352.379) radius 12
  line L0 (-0.1074, -0.221) -> (-0.1074, 514.979)
  line L1 (-0.1074, 514.979) -> (-507.9074, 514.979)
  line L2 (-507.9074, 514.979) -> (-507.9074, -0.221)
  line L3 (-507.9074, -0.221) -> (-0.1074, -0.221)
  circle A117 centre (-50.1074, 464.979) radius 7.5
  dimension "d283" = 15
  dimension "d284" = 50
  dimension "d285" = 50
  measures "d283" diameter of A117
  measures "d284" distance of L0 A117.centre
  measures "d285" distance of L1 A117.centre
extrude "Extrusion28" cut sketch "Skizze25" against normal blind 4 contours A117
